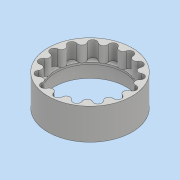
# Autodesk Inventor part: eq_Outer_main
Saved by Autodesk Inventor 2020.2 (Build 242310000, 310)
## iProperties
Created: 2018-11-04
Part Number: eq_Outer_main
Material: Allgemein
Document SubType Name: Modeling
Designer: paulg
Density: 1 g/cm^3
Appearance: Vorgabe
Author: paulg
Autodesk Inventor part; units mm, degrees
ref_plane "YZ Plane" through (0, 0, 0) normal (1, 0, 0) x (0, 1, 0)
ref_plane "XZ Plane" through (0, 0, 0) normal (0, 1, 0) x (-1, 0, 0)
ref_plane "XY Plane" through (0, 0, 0) normal (0, 0, 1) x (1, 0, 0)
sketch "Sketch1" plane through (0, 0, 0) normal (0, 0, 1) x (1, 0, 0)
  circle A0 centre (0, 0) radius 21.5
  line L0 (0, 0) -> (19.15, 0) construction
  circle A1 centre (19.15, 0) radius 2
  circle A2 centre (17.9464, 3.8146) radius 2
  circle A3 centre (0, 0) radius 18.646
  circle A4 centre (0, 0) radius 19.15 construction
  line L1 (17.9464, 3.8146) -> (34.7797, 7.3927) construction
  line L2 (-32.7559, 0) -> (46.0357, 0) construction
  point P0 (18.5482, 1.9073)
  point P1 (18.5482, -1.9073)
  point P2 (17.7204, 5.8018)
  dimension "d2" = 4
  dimension "d12" = 4
  dimension "d0" = 43
  dimension "d1" = 19.15
  dimension "d55" = 12
  constraints: 4 coincident, 4 end point, 1 centre point, 1 horizontal, 1 horizontal alignment, 12 other
  measures "d0" diameter of A0
  measures "d1" distance of L0.start L0.end
  measures "d55" angle of L2 L1
extrude "Extrusion1" add sketch "Sketch1" along normal blind 8 contours A0 | A1 A3 | A3 A2 picked at (19.405, -0.5136) picked at (18.7809, 4.0132)
extrude "Extrusion14" add sketch "Sketch1" along normal blind 8 separate body contours A1 A3 | A3 A1
pattern_circular "Runde Anordnung4" count 15 over 360 about axis through (0, 0, -10) along (0, 0, 1) of "Extrusion14" bodies 2
combine bodies "Kombinieren4" operation type add bodies to combine 1 2
extrude "Extrusion15" add sketch "Sketch1" along normal blind 8 separate body contours A3 A2 | A2 A3
pattern_circular "Runde Anordnung5" count 15 over 360 about axis through (0, 0, -10) along (0, 0, 1) of "Extrusion15" bodies 3
combine bodies "Kombinieren5" operation type subtract main body 1 bodies to subtract 3
sketch "Sketch4" plane through (0, 0, 0) normal (0, 0, -1) x (-1, 0, 0)
  circle A0 centre (0, 0) radius 17.5
  arc A1 (-18.5482, -1.9073) -> (-18.5482, 1.9073) centre (-19.15, 0) ccw projected
  arc A2 (-16.1689, -9.2867) -> (-17.7204, -5.8018) centre (-17.4944, -7.789) ccw projected
  arc A3 (-10.9938, -15.0602) -> (-13.8286, -12.5078) centre (-12.8139, -14.2312) ccw projected
  arc A4 (-3.9177, -18.2298) -> (-7.5457, -17.051) centre (-5.9177, -18.2127) ccw projected
  arc A5 (3.8357, -18.2472) -> (0.0419, -18.646) centre (2.0017, -19.0451) ccw projected
  arc A6 (10.9259, -15.1096) -> (7.6223, -17.0169) centre (9.575, -16.5844) ccw projected
  arc A7 (16.1269, -9.3593) -> (13.8847, -12.4454) centre (15.4927, -11.2561) ccw projected
  arc A8 (18.5394, -1.9908) -> (17.7463, -5.722) centre (18.7315, -3.9815) ccw projected
  arc A9 (17.7463, 5.722) -> (18.5394, 1.9908) centre (18.7315, 3.9815) ccw projected
  arc A10 (13.8847, 12.4454) -> (16.1269, 9.3593) centre (15.4927, 11.2561) ccw projected
  arc A11 (7.6223, 17.0169) -> (10.9259, 15.1096) centre (9.575, 16.5844) ccw projected
  arc A12 (0.0419, 18.646) -> (3.8357, 18.2472) centre (2.0017, 19.0451) ccw projected
  arc A13 (-7.5457, 17.051) -> (-3.9177, 18.2298) centre (-5.9177, 18.2127) ccw projected
  arc A14 (-13.8286, 12.5078) -> (-10.9938, 15.0602) centre (-12.8139, 14.2312) ccw projected
  arc A15 (-17.7204, 5.8018) -> (-16.1689, 9.2867) centre (-17.4944, 7.789) ccw projected
  arc A16 (-17.7204, 5.8018) -> (-18.5482, 1.9073) centre (-17.9464, 3.8146) ccw projected
  circle A17 centre (0, 0) radius 21.5 projected
  arc A18 (-13.8286, 12.5078) -> (-16.1689, 9.2867) centre (-14.8433, 10.7843) ccw projected
  arc A19 (-7.5457, 17.051) -> (-10.9938, 15.0602) centre (-9.1737, 15.8893) ccw projected
  arc A20 (0.0419, 18.646) -> (-3.9177, 18.2298) centre (-1.9178, 18.2468) ccw projected
  arc A21 (7.6223, 17.0169) -> (3.8357, 18.2472) centre (5.6696, 17.4494) ccw projected
  arc A22 (13.8847, 12.4454) -> (10.9259, 15.1096) centre (12.2768, 13.6347) ccw projected
  arc A23 (17.7463, 5.722) -> (16.1269, 9.3593) centre (16.7611, 7.4625) ccw projected
  arc A24 (18.5394, -1.9908) -> (18.5394, 1.9908) centre (18.3474, 0) ccw projected
  arc A25 (16.1269, -9.3593) -> (17.7463, -5.722) centre (16.7611, -7.4625) ccw projected
  arc A26 (10.9259, -15.1096) -> (13.8847, -12.4454) centre (12.2768, -13.6347) ccw projected
  arc A27 (3.8357, -18.2472) -> (7.6223, -17.0169) centre (5.6696, -17.4494) ccw projected
  arc A28 (-3.9177, -18.2298) -> (0.0419, -18.646) centre (-1.9178, -18.2468) ccw projected
  arc A29 (-10.9938, -15.0602) -> (-7.5457, -17.051) centre (-9.1737, -15.8893) ccw projected
  arc A30 (-16.1689, -9.2867) -> (-13.8286, -12.5078) centre (-14.8433, -10.7843) ccw projected
  arc A31 (-18.5482, -1.9073) -> (-17.7204, -5.8018) centre (-17.9464, -3.8146) ccw projected
  dimension "d19" = 35
  constraints: 1 centre point
  measures "d19" diameter of A0
extrude "Extrusion4" add sketch "Sketch4" along normal blind 1 contours A0 A9 A24 A8 | A0 A10 A23 A9 | A8 A25 A7 A0 | A0 A11 A22 A10 | A7 A26 A6 A0 | A0 A12 A21 A11 | A6 A27 A5 A0 | A0 A13 A20 A12 | A5 A28 A4 A0 | A0 A14 A19 A13 | A4 A29 A3 A0 | A0 A15 A18 A14 | A3 A30 A2 A0 | A0 A1 A16 A15 | A2 A31 A1 A0 | A17 bodies 1
sketch "Sketch5" plane through (0, 0, -1) normal (0, 0, -1) x (-1, 0, 0)
  circle A0 centre (0, 0) radius 18.65
  circle A1 centre (0, 0) radius 21.5 projected
  dimension "d22" = 37.3
  constraints: 1 centre point
  measures "d22" diameter of A0
extrude "Extrusion5" add sketch "Sketch5" along normal blind 7 bodies 1
equation "\"d2\" = 2 * Rr_"
equation "\"R_\" = 19"
equation "\"Rr_\" = 2"
equation "\"E_\" = 1"
equation "\"Ri\" = 11.75"
equation "\"Rli\" = 15"
equation "\"Rla\" = 18.5"
equation "\"Ra\" = 21.5"
equation "\"Rsi\" = 5"
equation "\"Rsa\" = 7.5"
equation "\"Rca\" = 7"
equation "\"Ras\" = 1"
equation "\"Rci\" = 5"
equation "\"Rea\" = 3.5"
equation "\"Rei\" = 2"
body "Solid1"
